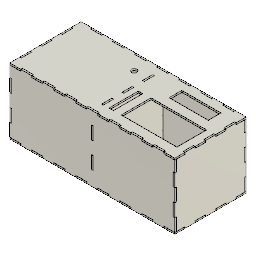
Final Enclosure (Autodesk Fusion 360 design; units mm, degrees)
Autodesk Fusion 360 part; units mm, degrees
note: some values were not read from the file. Chosen so that the rebuilt part matches the saved one: which bodies a step acts on.
(part 1 of 2)
sketch "Bottom Panel Profile Sketch" plane through (0, 0, 0) normal (0, 0, 1) x (1, 0, 0) in component "Main Box"
  line L0 (0, 0) -> (300, 0)
  line L1 (300, 0) -> (300, 130)
  line L2 (300, 130) -> (0, 130)
  line L3 (0, 130) -> (0, 0)
  dimension "d21" = 300
  dimension "d22" = 130
  constraint horizontal L0
  constraint vertical L1
  constraint horizontal L2
  constraint vertical L3
  constraint coincident L0.start L3.end
  measures "d21" distance of L0.start L0.end
  measures "d22" distance of L0.start L2.end
extrude "Bottom Panel Extrude" add sketch "Bottom Panel Profile Sketch" along normal blind 3 makes body 1 in component "Main Box"
sketch "Bottom Panel Front Fingers Sketch" plane through (0, 0, 0) normal (0, -1, 0) x (1, 0, 0) in component "Main Box"
  line L0 (0, 0) -> (300, 0)
  line L1 (300, 0) -> (300, 3)
  line L2 (300, 3) -> (0, 3)
  line L3 (0, 3) -> (0, 0)
  line L4 (150, 3) -> (150, 0) construction
  line L5 (20, 1.5) -> (280, 1.5) construction
  line L6 (20, 0) -> (40, 0)
  line L7 (40, 0) -> (40, 3)
  line L8 (40, 3) -> (20, 3)
  line L9 (20, 3) -> (20, 0)
  dimension "d25" = 20
  dimension "d26" = 260
  constraint midpoint L2 L4.start
  constraint midpoint L0 L4.end
  constraint perpendicular L4 L5
  constraint midpoint L4 L5
  constraint horizontal L6
  constraint vertical L7
  constraint horizontal L8
  constraint vertical L9
  constraint coincident L2 L7.end
  constraint coincident L0 L6.start
  constraint coincident L5.start L9
  measures "d25" horizontal distance of L7.end L8.end
  measures "d26" horizontal distance of L5.start L5.end
extrude "Bottom Panel Front Finger Extrude" cut sketch "Bottom Panel Front Fingers Sketch" against normal blind 3 contours L0 L2 L6 L7 L8 L9 bodies 1 in component "Main Box"
pattern_linear "Bottom Panel Length Fingers Pattern" count 7 spacing 40 along (1, 0, 0) count 2 spacing 127 along (0, 1, 0) of "Bottom Panel Front Finger Extrude" in component "Main Box"
sketch "Bottom Panel Left Fingers Sketch" plane through (0, 0, 0) normal (-1, 0, 0) x (0, -1, 0) in component "Main Box"
  line L0 (-130, 0) -> (0, 0)
  line L1 (0, 0) -> (0, 3)
  line L2 (0, 3) -> (-130, 3)
  line L3 (-130, 3) -> (-130, 0)
  line L4 (-65, 3) -> (-65, 0) construction
  line L5 (-111.4286, 1.5) -> (-18.5714, 1.5) construction
  line L6 (-18.5714, 0) -> (-37.1429, 0)
  line L7 (-37.1429, 0) -> (-37.1429, 3)
  line L8 (-37.1429, 3) -> (-18.5714, 3)
  line L9 (-18.5714, 3) -> (-18.5714, 0)
  dimension "d33" = 18.5714
  dimension "d34" = 92.8571
  constraint midpoint L2 L4.start
  constraint midpoint L0 L4.end
  constraint perpendicular L4 L5
  constraint midpoint L4 L5
  constraint horizontal L6
  constraint vertical L7
  constraint horizontal L8
  constraint vertical L9
  constraint coincident L2 L7.end
  constraint coincident L0 L6.start
  constraint coincident L5.end L9
  measures "d33" horizontal distance of L6.start L6.end
  measures "d34" horizontal distance of L5.start L5.end
extrude "Bottom Panel Left Finger Extrude" cut sketch "Bottom Panel Left Fingers Sketch" against normal blind 3 contours L0 L2 L6 L7 L8 L9 bodies 1 in component "Main Box"
pattern_linear "Bottom Panel Width Fingers Pattern" count 3 spacing 37.1429 along (0, 1, 0) count 3 spacing 148.5 along (1, 0, 0) of "Bottom Panel Left Finger Extrude" in component "Main Box"
sketch "Front Panel Profile Sketch" plane through (0, 0, 0) normal (0, 1, 0) x (1, 0, 0) in component "Main Box"
  line L0 (0, 0) -> (300, 0)
  line L1 (300, 0) -> (300, -120)
  line L2 (300, -120) -> (0, -120)
  line L3 (0, -120) -> (0, 0)
  dimension "d41" = 300
  dimension "d42" = 120
  constraint horizontal L0
  constraint vertical L1
  constraint horizontal L2
  constraint vertical L3
  constraint coincident L0.start L3.end
  measures "d41" distance of L0.start L0.end
  measures "d42" distance of L0.start L2.end
extrude "Front Panel Extrude" add sketch "Front Panel Profile Sketch" along normal blind 3 separate body makes body 2 in component "Main Box"
combine "Front Panel Combine" operation cut target body 2 tool bodies 1 keep tools in component "Main Box"
sketch "Front Panel Left Fingers Sketch" plane through (0, 0, 0) normal (0, -1, 0) x (1, 0, 0) in component "Main Box"
  line L0 (300, 3) -> (300, 120)
  line L1 (300, 120) -> (0, 120)
  line L2 (0, 120) -> (0, 3)
  line L3 (280, 3) -> (300, 3)
  line L4 (20, 3) -> (20, 0)
  line L5 (20, 0) -> (40, 0)
  line L6 (40, 0) -> (40, 3)
  line L7 (40, 3) -> (60, 3)
  line L8 (0, 61.5) -> (3, 61.5) construction
  line L9 (1.5, 96.6) -> (1.5, 26.4) construction
  line L10 (0, 26.4) -> (3, 26.4)
  line L11 (3, 26.4) -> (3, 49.8)
  line L12 (3, 49.8) -> (0, 49.8)
  line L13 (0, 49.8) -> (0, 26.4)
  line L14 (60, 3) -> (60, 0)
  line L15 (60, 0) -> (80, 0)
  line L16 (80, 0) -> (80, 3)
  line L17 (80, 3) -> (100, 3)
  line L18 (100, 3) -> (100, 0)
  line L19 (100, 0) -> (120, 0)
  line L20 (120, 0) -> (120, 3)
  line L21 (120, 3) -> (140, 3)
  line L22 (140, 3) -> (140, 0)
  line L23 (140, 0) -> (160, 0)
  line L24 (160, 0) -> (160, 3)
  line L25 (160, 3) -> (180, 3)
  line L26 (180, 3) -> (180, 0)
  line L27 (180, 0) -> (200, 0)
  line L28 (200, 0) -> (200, 3)
  line L29 (200, 3) -> (220, 3)
  line L30 (220, 3) -> (220, 0)
  line L31 (220, 0) -> (240, 0)
  line L32 (240, 0) -> (240, 3)
  line L33 (240, 3) -> (260, 3)
  line L34 (260, 3) -> (260, 0)
  line L35 (260, 0) -> (280, 0)
  line L36 (280, 0) -> (280, 3)
  line L37 (0, 3) -> (20, 3)
  dimension "d45" = 3
  dimension "d46" = 23.4
  dimension "d47" = 70.2
  constraint midpoint L2 L8.start
  constraint perpendicular L2 L8
  constraint perpendicular L8 L9
  constraint midpoint L8 L9
  constraint horizontal L10
  constraint vertical L11
  constraint horizontal L12
  constraint vertical L13
  constraint coincident L2 L10.start
  constraint coincident L9.end L10
  constraint coincident L8.end L11
  measures "d45" distance of L8.start L8.end
  measures "d46" vertical distance of L10.start L12.end
  measures "d47" vertical distance of L9.start L9.end
extrude "Front Panel Left Fingers Extrude" cut sketch "Front Panel Left Fingers Sketch" against normal blind 3 contours L2 L10 L11 L12 L13 bodies 2 in component "Main Box"
pattern_linear "Front Panel Height Fingers Pattern" count 2 spacing 46.8 along (0, 0, 1) count 3 spacing 148.5 along (1, 0, 0) of "Front Panel Left Fingers Extrude" in component "Main Box"
pattern_linear "Front Panel Pattern" count 2 spacing 127 along (0, 1, 0) of bodies 2 makes body 3 in component "Main Box"
sketch "Left Panel Profile Sketch" plane through (0, 0, 0) normal (1, 0, 0) x (0, 1, 0) in component "Main Box"
  line L0 (0, 0) -> (130, 0)
  line L1 (130, 0) -> (130, 120)
  line L2 (130, 120) -> (0, 120)
  line L3 (0, 120) -> (0, 0)
  dimension "d58" = 130
  dimension "d59" = 120
  constraint horizontal L0
  constraint vertical L1
  constraint horizontal L2
  constraint vertical L3
  constraint coincident L0.start L3.end
  measures "d58" distance of L0.start L0.end
  measures "d59" distance of L0.start L2.end
extrude "Left Panel Extrude" add sketch "Left Panel Profile Sketch" along normal blind 3 separate body makes body 4 in component "Main Box"
sketch "Left Panel Front Fingers Sketch" plane through (0, 0, 0) normal (0, -1, 0) x (1, 0, 0) in component "Main Box"
  line L0 (0, 120) -> (0, 0)
  line L1 (0, 0) -> (3, 0)
  line L2 (3, 0) -> (3, 120)
  line L3 (3, 120) -> (0, 120)
  line L4 (0, 120) -> (3, 120)
  line L5 (3, 120) -> (3, 96.6)
  line L6 (3, 96.6) -> (0, 96.6)
  line L7 (0, 96.6) -> (0, 120)
  dimension "d72" = 23.4
  constraint horizontal L4
  constraint vertical L5
  constraint horizontal L6
  constraint vertical L7
  constraint coincident L2 L5.end
  constraint coincident L0.start L3.end
  measures "d72" vertical distance of L0.start L6.end
extrude "Left Panel Front Fingers Extrude" cut sketch "Left Panel Front Fingers Sketch" against normal blind 3 contours L0 L2 L3 L4 L5 L6 L7 bodies 4 in component "Main Box"
pattern_linear "Left Panel Slots Pattern" count 2 spacing 127 along (0, 1, 0) of "Left Panel Front Fingers Extrude" in component "Main Box"
combine "Left Panel Combine" operation cut target body 4 tool bodies 3 1 2 keep tools in component "Main Box"
pattern_linear "Left Panel Pattern" count 3 spacing 148.5 along (1, 0, 0) of bodies 4 makes body 5 at (300, 61.9048, 49.8) makes body 6 at (151.5, 61.9048, 49.8) in component "Main Box"
sketch "Sketch1" plane through (0, 0, 0) normal (0, -1, 0) x (1, 0, 0)
  line L0 (297, 49.8) -> (300, 49.8)
  line L1 (300, 96.6) -> (300, 120)
  line L2 (300, 120) -> (0, 120)
  line L3 (0, 120) -> (0, 96.6)
  line L4 (0, 49.8) -> (3, 49.8)
  line L5 (3, 49.8) -> (3, 26.4)
  line L6 (3, 26.4) -> (0, 26.4)
  line L7 (0, 26.4) -> (0, 3)
  line L8 (0, 3) -> (20, 3)
  line L9 (20, 3) -> (20, 0)
  line L10 (20, 0) -> (40, 0)
  line L11 (40, 0) -> (40, 3)
  line L12 (40, 3) -> (60, 3)
  line L13 (60, 3) -> (60, 0)
  line L14 (60, 0) -> (80, 0)
  line L15 (80, 0) -> (80, 3)
  line L16 (80, 3) -> (100, 3)
  line L17 (100, 3) -> (100, 0)
  line L18 (100, 0) -> (120, 0)
  line L19 (120, 0) -> (120, 3)
  line L20 (120, 3) -> (140, 3)
  line L21 (140, 3) -> (140, 0)
  line L22 (140, 0) -> (160, 0)
  line L23 (160, 0) -> (160, 3)
  line L24 (160, 3) -> (180, 3)
  line L25 (180, 3) -> (180, 0)
  line L26 (180, 0) -> (200, 0)
  line L27 (200, 0) -> (200, 3)
  line L28 (200, 3) -> (220, 3)
  line L29 (220, 3) -> (220, 0)
  line L30 (220, 0) -> (240, 0)
  line L31 (240, 0) -> (240, 3)
  line L32 (240, 3) -> (260, 3)
  line L33 (260, 3) -> (260, 0)
  line L34 (260, 0) -> (280, 0)
  line L35 (280, 0) -> (280, 3)
  line L36 (280, 3) -> (300, 3)
  line L37 (300, 3) -> (300, 26.4)
  line L38 (300, 26.4) -> (297, 26.4)
  line L39 (297, 26.4) -> (297, 49.8)
  line L40 (151.5, 26.4) -> (148.5, 26.4)
  line L41 (148.5, 26.4) -> (148.5, 49.8)
  line L42 (148.5, 49.8) -> (151.5, 49.8)
  line L43 (151.5, 49.8) -> (151.5, 26.4)
  line L44 (297, 96.6) -> (300, 96.6)
  line L45 (0, 96.6) -> (3, 96.6)
  line L46 (3, 96.6) -> (3, 73.2)
  line L47 (3, 73.2) -> (0, 73.2)
  line L48 (0, 73.2) -> (0, 49.8)
  line L49 (300, 49.8) -> (300, 73.2)
  line L50 (300, 73.2) -> (297, 73.2)
  line L51 (297, 73.2) -> (297, 96.6)
  line L52 (151.5, 73.2) -> (148.5, 73.2)
  line L53 (148.5, 96.6) -> (151.5, 96.6)
extrude "Extrude1" add 1 faces at (102.8333, 68.0952, 3) along direction (0, 0, 1) blind 117 separate body on bodies 1 makes body 7
extrude "Extrude2" add 1 faces at (102.8333, 68.0952, 3) along direction (0, 0, 1) blind 3 from surface at 114 separate body on bodies 1 makes body 8
combine "Combine3" operation cut target body 4 tool bodies 8 keep tools in component "Main Box"
combine "Combine4" operation cut target body 2 tool bodies 8 keep tools in component "Main Box"
combine "Combine5" operation cut target body 5 tool bodies 8 keep tools in component "Main Box"
combine "Combine6" operation cut target body 3 tool bodies 8 keep tools in component "Main Box"
combine "Combine7" operation cut target body 6 tool bodies 8 keep tools in component "Main Box"
sketch "Sketch12" plane through (0, 0, 120) normal (0, 0, 1) x (-1, 0, 0)
  line L0 (-151.5, -18.5714) -> (-148.5, -18.5714)
  line L1 (-148.5, -18.5714) -> (-148.5, -37.1429)
  line L2 (-148.5, -37.1429) -> (-151.5, -37.1429)
  line L3 (-151.5, -37.1429) -> (-151.5, -18.5714)
  line L4 (-151.5, -55.7143) -> (-148.5, -55.7143)
  line L5 (-148.5, -55.7143) -> (-148.5, -74.2857)
  line L6 (-148.5, -74.2857) -> (-151.5, -74.2857)
  line L7 (-151.5, -74.2857) -> (-151.5, -55.7143)
  line L8 (-151.5, -92.8571) -> (-148.5, -92.8571)
  line L9 (-148.5, -92.8571) -> (-148.5, -111.4286)
  line L10 (-148.5, -111.4286) -> (-151.5, -111.4286)
  line L11 (-151.5, -111.4286) -> (-151.5, -92.8571)
  line L12 (-300, -92.8571) -> (-297, -92.8571)
  line L13 (-297, -92.8571) -> (-297, -111.4286)
  line L14 (-297, -111.4286) -> (-300, -111.4286)
  line L15 (-300, -111.4286) -> (-300, -130)
  line L16 (-300, -130) -> (-280, -130)
  line L17 (-280, -130) -> (-280, -127)
  line L18 (-280, -127) -> (-260, -127)
  line L19 (-260, -127) -> (-260, -130)
  line L20 (-260, -130) -> (-240, -130)
  line L21 (-240, -130) -> (-240, -127)
  line L22 (-240, -127) -> (-220, -127)
  line L23 (-220, -127) -> (-220, -130)
  line L24 (-220, -130) -> (-200, -130)
  line L25 (-200, -130) -> (-200, -127)
  line L26 (-200, -127) -> (-180, -127)
  line L27 (-180, -127) -> (-180, -130)
  line L28 (-180, -130) -> (-160, -130)
  line L29 (-160, -130) -> (-160, -127)
  line L30 (-160, -127) -> (-140, -127)
  line L31 (-140, -127) -> (-140, -130)
  line L32 (-140, -130) -> (-120, -130)
  line L33 (-120, -130) -> (-120, -127)
  line L34 (-120, -127) -> (-100, -127)
  line L35 (-100, -127) -> (-100, -130)
  line L36 (-100, -130) -> (-80, -130)
  line L37 (-80, -130) -> (-80, -127)
  line L38 (-80, -127) -> (-60, -127)
  line L39 (-60, -127) -> (-60, -130)
  line L40 (-60, -130) -> (-40, -130)
  line L41 (-40, -130) -> (-40, -127)
  line L42 (-40, -127) -> (-20, -127)
  line L43 (-20, -127) -> (-20, -130)
  line L44 (-20, -130) -> (0, -130)
  line L45 (0, -130) -> (0, -111.4286)
  line L46 (0, -111.4286) -> (-3, -111.4286)
  line L47 (-3, -111.4286) -> (-3, -92.8571)
  line L48 (-3, -92.8571) -> (0, -92.8571)
  line L49 (0, -92.8571) -> (0, -74.2857)
  line L50 (0, -74.2857) -> (-3, -74.2857)
  line L51 (-3, -74.2857) -> (-3, -55.7143)
  line L52 (-3, -55.7143) -> (0, -55.7143)
  line L53 (0, -55.7143) -> (0, -37.1429)
  line L54 (0, -37.1429) -> (-3, -37.1429)
  line L55 (-3, -37.1429) -> (-3, -18.5714)
  line L56 (-3, -18.5714) -> (0, -18.5714)
  line L57 (0, -18.5714) -> (0, 0)
  line L58 (0, 0) -> (-20, 0)
  line L59 (-20, 0) -> (-20, -3)
  line L60 (-20, -3) -> (-40, -3)
  line L61 (-40, -3) -> (-40, 0)
  line L62 (-40, 0) -> (-60, 0)
  line L63 (-60, 0) -> (-60, -3)
  line L64 (-60, -3) -> (-80, -3)
  line L65 (-80, -3) -> (-80, 0)
  line L66 (-80, 0) -> (-100, 0)
  line L67 (-100, 0) -> (-100, -3)
  line L68 (-100, -3) -> (-120, -3)
  line L69 (-120, -3) -> (-120, 0)
  line L70 (-120, 0) -> (-140, 0)
  line L71 (-140, 0) -> (-140, -3)
  line L72 (-140, -3) -> (-160, -3)
  line L73 (-160, -3) -> (-160, 0)
  line L74 (-160, 0) -> (-180, 0)
  line L75 (-180, 0) -> (-180, -3)
  line L76 (-180, -3) -> (-200, -3)
  line L77 (-200, -3) -> (-200, 0)
  line L78 (-200, 0) -> (-220, 0)
  line L79 (-220, 0) -> (-220, -3)
  line L80 (-220, -3) -> (-240, -3)
  line L81 (-240, -3) -> (-240, 0)
  line L82 (-240, 0) -> (-260, 0)
  line L83 (-260, 0) -> (-260, -3)
  line L84 (-260, -3) -> (-280, -3)
  line L85 (-280, -3) -> (-280, 0)
  line L86 (-280, 0) -> (-300, 0)
  line L87 (-300, 0) -> (-300, -18.5714)
  line L88 (-300, -18.5714) -> (-297, -18.5714)
  line L89 (-297, -18.5714) -> (-297, -37.1429)
  line L90 (-297, -37.1429) -> (-300, -37.1429)
  line L91 (-300, -37.1429) -> (-300, -55.7143)
  line L92 (-300, -55.7143) -> (-297, -55.7143)
  line L93 (-297, -55.7143) -> (-297, -74.2857)
  line L94 (-297, -74.2857) -> (-300, -74.2857)
  line L95 (-300, -74.2857) -> (-300, -92.8571)
  circle A0 centre (-125.8569, -100.5311) radius 5
  line L96 (-199.7569, -113.0322) -> (-270.7569, -113.0322)
  line L97 (-270.7569, -113.0322) -> (-270.7569, -90.0322)
  line L98 (-270.7569, -90.0322) -> (-199.7569, -90.0322)
  line L99 (-199.7569, -90.0322) -> (-199.7569, -113.0322)
  line L100 (-183.4296, -73.3855) -> (-284.4296, -73.3855)
  line L101 (-284.4296, -73.3855) -> (-284.4296, -19.3855)
  line L102 (-284.4296, -19.3855) -> (-183.4296, -19.3855)
  line L103 (-183.4296, -19.3855) -> (-183.4296, -73.3855)
  line L104 (-161.4021, -72.4445) -> (-169.4021, -72.4445)
  line L105 (-169.4021, -72.4445) -> (-169.4021, -19.1021)
  line L106 (-169.4021, -19.1021) -> (-161.4021, -19.1021)
  line L107 (-161.4021, -19.1021) -> (-161.4021, -72.4445)
  dimension "d109" = 10
  dimension "d110" = 71
  dimension "d111" = 23
  dimension "d112" = 101
  dimension "d113" = 54
  dimension "d114" = 8
  constraint horizontal L96
  constraint vertical L97
  constraint horizontal L98
  constraint vertical L99
  constraint horizontal L100
  constraint vertical L101
  constraint horizontal L102
  constraint vertical L103
  constraint horizontal L104
  constraint vertical L105
  constraint horizontal L106
  constraint vertical L107
  measures "d109" diameter of A0
  measures "d110" distance of L96.start L96.end
  measures "d111" distance of L96.start L98.end
  measures "d112" distance of L100.start L100.end
  measures "d113" distance of L100.start L102.end
  measures "d114" distance of L104.start L104.end
extrude "Extrude4" cut sketch "Sketch12" against normal blind 3 contours A0 | L96 L97 L98 L99 | L100 L101 L102 L103 | L104 L105 L106 L107 bodies 8
sketch "Sketch14" plane through (151.5, 0, 0) normal (1, 0, 0) x (0, 1, 0)
  line L0 (18.5714, 117) -> (3, 117)
  line L1 (3, 117) -> (3, 96.6)
  line L2 (3, 96.6) -> (0, 96.6)
  line L3 (0, 96.6) -> (0, 73.2)
  line L4 (0, 73.2) -> (3, 73.2)
  line L5 (3, 73.2) -> (3, 49.8)
  line L6 (3, 49.8) -> (0, 49.8)
  line L7 (0, 49.8) -> (0, 26.4)
  line L8 (0, 26.4) -> (3, 26.4)
  line L9 (3, 26.4) -> (3, 3)
  line L10 (3, 3) -> (18.5714, 3)
  line L11 (18.5714, 3) -> (18.5714, 0)
  line L12 (18.5714, 0) -> (37.1429, 0)
  line L13 (37.1429, 0) -> (37.1429, 3)
  line L14 (37.1429, 3) -> (55.7143, 3)
  line L15 (55.7143, 3) -> (55.7143, 0)
  line L16 (55.7143, 0) -> (74.2857, 0)
  line L17 (74.2857, 0) -> (74.2857, 3)
  line L18 (74.2857, 3) -> (92.8571, 3)
  line L19 (92.8571, 3) -> (92.8571, 0)
  line L20 (92.8571, 0) -> (111.4286, 0)
  line L21 (111.4286, 0) -> (111.4286, 3)
  line L22 (111.4286, 3) -> (127, 3)
  line L23 (127, 3) -> (127, 26.4)
  line L24 (127, 26.4) -> (130, 26.4)
  line L25 (130, 26.4) -> (130, 49.8)
  line L26 (130, 49.8) -> (127, 49.8)
  line L27 (127, 49.8) -> (127, 73.2)
  line L28 (127, 73.2) -> (130, 73.2)
  line L29 (130, 73.2) -> (130, 96.6)
  line L30 (130, 96.6) -> (127, 96.6)
  line L31 (127, 96.6) -> (127, 117)
  line L32 (127, 117) -> (111.4286, 117)
  line L33 (111.4286, 117) -> (111.4286, 120)
  line L34 (111.4286, 120) -> (92.8571, 120)
  line L35 (92.8571, 120) -> (92.8571, 117)
  line L36 (92.8571, 117) -> (74.2857, 117)
  line L37 (74.2857, 117) -> (74.2857, 120)
  line L38 (74.2857, 120) -> (55.7143, 120)
  line L39 (55.7143, 120) -> (55.7143, 117)
  line L40 (55.7143, 117) -> (37.1429, 117)
  line L41 (37.1429, 117) -> (37.1429, 120)
  line L42 (37.1429, 120) -> (18.5714, 120)
  line L43 (18.5714, 120) -> (18.5714, 117)
  circle A0 centre (63.791, 90.8075) radius 9.4231
extrude "Extrude10" [rolled back] taper angle 0 in component "Main Box"
sketch "FRONTBACK" plane through (0, 130, 0) normal (0, 1, 0) x (-1, 0, 0)
  line L0 (0, 117) -> (-20, 117)
  line L1 (-20, 117) -> (-20, 120)
  line L2 (-20, 120) -> (-40, 120)
  line L3 (-40, 120) -> (-40, 117)
  line L4 (-40, 117) -> (-60, 117)
  line L5 (-60, 117) -> (-60, 120)
  line L6 (-60, 120) -> (-80, 120)
  line L7 (-80, 120) -> (-80, 117)
  line L8 (-80, 117) -> (-100, 117)
  line L9 (-100, 117) -> (-100, 120)
  line L10 (-100, 120) -> (-120, 120)
  line L11 (-120, 120) -> (-120, 117)
  line L12 (-120, 117) -> (-140, 117)
  line L13 (-140, 117) -> (-140, 120)
  line L14 (-140, 120) -> (-160, 120)
  line L15 (-160, 120) -> (-160, 117)
  line L16 (-160, 117) -> (-180, 117)
  line L17 (-180, 117) -> (-180, 120)
  line L18 (-180, 120) -> (-200, 120)
  line L19 (-200, 120) -> (-200, 117)
  line L20 (-200, 117) -> (-220, 117)
  line L21 (-220, 117) -> (-220, 120)
  line L22 (-220, 120) -> (-240, 120)
  line L23 (-240, 120) -> (-240, 117)
  line L24 (-240, 117) -> (-260, 117)
  line L25 (-260, 117) -> (-260, 120)
  line L26 (-260, 120) -> (-280, 120)
  line L27 (-280, 120) -> (-280, 117)
  line L28 (-280, 117) -> (-300, 117)
  line L29 (-300, 117) -> (-300, 96.6)
  line L30 (-300, 96.6) -> (-297, 96.6)
  line L31 (-297, 96.6) -> (-297, 73.2)
  line L32 (-297, 73.2) -> (-300, 73.2)
  line L33 (-300, 73.2) -> (-300, 49.8)
  line L34 (-300, 49.8) -> (-297, 49.8)
  line L35 (-297, 49.8) -> (-297, 26.4)
  line L36 (-297, 26.4) -> (-300, 26.4)
  line L37 (-300, 26.4) -> (-300, 3)
  line L38 (-300, 3) -> (-280, 3)
  line L39 (-280, 3) -> (-280, 0)
  line L40 (-280, 0) -> (-260, 0)
  line L41 (-260, 0) -> (-260, 3)
  line L42 (-260, 3) -> (-240, 3)
  line L43 (-240, 3) -> (-240, 0)
  line L44 (-240, 0) -> (-220, 0)
  line L45 (-220, 0) -> (-220, 3)
  line L46 (-220, 3) -> (-200, 3)
  line L47 (-200, 3) -> (-200, 0)
  line L48 (-200, 0) -> (-180, 0)
  line L49 (-180, 0) -> (-180, 3)
  line L50 (-180, 3) -> (-160, 3)
  line L51 (-160, 3) -> (-160, 0)
  line L52 (-160, 0) -> (-140, 0)
  line L53 (-140, 0) -> (-140, 3)
  line L54 (-140, 3) -> (-120, 3)
  line L55 (-120, 3) -> (-120, 0)
  line L56 (-120, 0) -> (-100, 0)
  line L57 (-100, 0) -> (-100, 3)
  line L58 (-100, 3) -> (-80, 3)
  line L59 (-80, 3) -> (-80, 0)
  line L60 (-80, 0) -> (-60, 0)
  line L61 (-60, 0) -> (-60, 3)
  line L62 (-60, 3) -> (-40, 3)
  line L63 (-40, 3) -> (-40, 0)
  line L64 (-40, 0) -> (-20, 0)
  line L65 (-20, 0) -> (-20, 3)
  line L66 (-20, 3) -> (0, 3)
  line L67 (0, 3) -> (0, 26.4)
  line L68 (0, 26.4) -> (-3, 26.4)
  line L69 (-3, 26.4) -> (-3, 49.8)
  line L70 (-3, 49.8) -> (0, 49.8)
  line L71 (0, 49.8) -> (0, 73.2)
  line L72 (0, 73.2) -> (-3, 73.2)
  line L73 (-3, 73.2) -> (-3, 96.6)
  line L74 (-3, 96.6) -> (0, 96.6)
  line L75 (0, 96.6) -> (0, 117)
  line L76 (-148.5, 73.2) -> (-151.5, 73.2)
  line L77 (-151.5, 73.2) -> (-151.5, 96.6)
  line L78 (-151.5, 96.6) -> (-148.5, 96.6)
  line L79 (-148.5, 96.6) -> (-148.5, 73.2)
  line L80 (-148.5, 26.4) -> (-151.5, 26.4)
  line L81 (-151.5, 26.4) -> (-151.5, 49.8)
  line L82 (-151.5, 49.8) -> (-148.5, 49.8)
  line L83 (-148.5, 49.8) -> (-148.5, 26.4)
sketch "LEFT RIGHT" plane through (300, 0, 0) normal (1, 0, 0) x (0, 1, 0)
  line L0 (18.5714, 117) -> (3, 117)
  line L1 (3, 117) -> (3, 96.6)
  line L2 (3, 96.6) -> (0, 96.6)
  line L3 (0, 96.6) -> (0, 73.2)
  line L4 (0, 73.2) -> (3, 73.2)
  line L5 (3, 73.2) -> (3, 49.8)
  line L6 (3, 49.8) -> (0, 49.8)
  line L7 (0, 49.8) -> (0, 26.4)
  line L8 (0, 26.4) -> (3, 26.4)
  line L9 (3, 26.4) -> (3, 3)
  line L10 (3, 3) -> (18.5714, 3)
  line L11 (18.5714, 3) -> (18.5714, 0)
  line L12 (18.5714, 0) -> (37.1429, 0)
  line L13 (37.1429, 0) -> (37.1429, 3)
  line L14 (37.1429, 3) -> (55.7143, 3)
  line L15 (55.7143, 3) -> (55.7143, 0)
  line L16 (55.7143, 0) -> (74.2857, 0)
  line L17 (74.2857, 0) -> (74.2857, 3)
  line L18 (74.2857, 3) -> (92.8571, 3)
  line L19 (92.8571, 3) -> (92.8571, 0)
  line L20 (92.8571, 0) -> (111.4286, 0)
  line L21 (111.4286, 0) -> (111.4286, 3)
  line L22 (111.4286, 3) -> (127, 3)
  line L23 (127, 3) -> (127, 26.4)
  line L24 (127, 26.4) -> (130, 26.4)
  line L25 (130, 26.4) -> (130, 49.8)
  line L26 (130, 49.8) -> (127, 49.8)
  line L27 (127, 49.8) -> (127, 73.2)
  line L28 (127, 73.2) -> (130, 73.2)
  line L29 (130, 73.2) -> (130, 96.6)
  line L30 (130, 96.6) -> (127, 96.6)
  line L31 (127, 96.6) -> (127, 117)
  line L32 (127, 117) -> (111.4286, 117)
  line L33 (111.4286, 117) -> (111.4286, 120)
  line L34 (111.4286, 120) -> (92.8571, 120)
  line L35 (92.8571, 120) -> (92.8571, 117)
  line L36 (92.8571, 117) -> (74.2857, 117)
  line L37 (74.2857, 117) -> (74.2857, 120)
  line L38 (74.2857, 120) -> (55.7143, 120)
  line L39 (55.7143, 120) -> (55.7143, 117)
  line L40 (55.7143, 117) -> (37.1429, 117)
  line L41 (37.1429, 117) -> (37.1429, 120)
  line L42 (37.1429, 120) -> (18.5714, 120)
  line L43 (18.5714, 120) -> (18.5714, 117)
sketch "MIDDLE PIECE" plane through (151.5, 0, 0) normal (1, 0, 0) x (0, 1, 0)
  circle A0 centre (63.791, 90.8075) radius 9.4231
  line L0 (18.5714, 117) -> (3, 117)
  line L1 (3, 117) -> (3, 96.6)
  line L2 (3, 96.6) -> (0, 96.6)
  line L3 (0, 96.6) -> (0, 73.2)
  line L4 (0, 73.2) -> (3, 73.2)
  line L5 (3, 73.2) -> (3, 49.8)
  line L6 (3, 49.8) -> (0, 49.8)
  line L7 (0, 49.8) -> (0, 26.4)
  line L8 (0, 26.4) -> (3, 26.4)
  line L9 (3, 26.4) -> (3, 3)
  line L10 (3, 3) -> (18.5714, 3)
  line L11 (18.5714, 3) -> (18.5714, 0)
  line L12 (18.5714, 0) -> (37.1429, 0)
  line L13 (37.1429, 0) -> (37.1429, 3)
  line L14 (37.1429, 3) -> (55.7143, 3)
  line L15 (55.7143, 3) -> (55.7143, 0)
  line L16 (55.7143, 0) -> (74.2857, 0)
  line L17 (74.2857, 0) -> (74.2857, 3)
  line L18 (74.2857, 3) -> (92.8571, 3)
  line L19 (92.8571, 3) -> (92.8571, 0)
  line L20 (92.8571, 0) -> (111.4286, 0)
  line L21 (111.4286, 0) -> (111.4286, 3)
  line L22 (111.4286, 3) -> (127, 3)
  line L23 (127, 3) -> (127, 26.4)
  line L24 (127, 26.4) -> (130, 26.4)
  line L25 (130, 26.4) -> (130, 49.8)
  line L26 (130, 49.8) -> (127, 49.8)
  line L27 (127, 49.8) -> (127, 73.2)
  line L28 (127, 73.2) -> (130, 73.2)
  line L29 (130, 73.2) -> (130, 96.6)
  line L30 (130, 96.6) -> (127, 96.6)
  line L31 (127, 96.6) -> (127, 117)
  line L32 (127, 117) -> (111.4286, 117)
  line L33 (111.4286, 117) -> (111.4286, 120)
  line L34 (111.4286, 120) -> (92.8571, 120)
  line L35 (92.8571, 120) -> (92.8571, 117)
  line L36 (92.8571, 117) -> (74.2857, 117)
  line L37 (74.2857, 117) -> (74.2857, 120)
  line L38 (74.2857, 120) -> (55.7143, 120)
  line L39 (55.7143, 120) -> (55.7143, 117)
  line L40 (55.7143, 117) -> (37.1429, 117)
  line L41 (37.1429, 117) -> (37.1429, 120)
  line L42 (37.1429, 120) -> (18.5714, 120)
  line L43 (18.5714, 120) -> (18.5714, 117)
sketch "BOTTOM" plane through (0, 0, 3) normal (0, 0, 1) x (-1, 0, 0)
  line L0 (-151.5, -18.5714) -> (-148.5, -18.5714)
  line L1 (-148.5, -18.5714) -> (-148.5, -37.1429)
  line L2 (-148.5, -37.1429) -> (-151.5, -37.1429)
  line L3 (-151.5, -37.1429) -> (-151.5, -18.5714)
  line L4 (-151.5, -55.7143) -> (-148.5, -55.7143)
  line L5 (-148.5, -55.7143) -> (-148.5, -74.2857)
  line L6 (-148.5, -74.2857) -> (-151.5, -74.2857)
  line L7 (-151.5, -74.2857) -> (-151.5, -55.7143)
  line L8 (-151.5, -92.8571) -> (-148.5, -92.8571)
  line L9 (-148.5, -92.8571) -> (-148.5, -111.4286)
  line L10 (-148.5, -111.4286) -> (-151.5, -111.4286)
  line L11 (-151.5, -111.4286) -> (-151.5, -92.8571)
  line L12 (-300, -92.8571) -> (-297, -92.8571)
  line L13 (-297, -92.8571) -> (-297, -111.4286)
  line L14 (-297, -111.4286) -> (-300, -111.4286)
  line L15 (-300, -111.4286) -> (-300, -130)
  line L16 (-300, -130) -> (-280, -130)
  line L17 (-280, -130) -> (-280, -127)
  line L18 (-280, -127) -> (-260, -127)
  line L19 (-260, -127) -> (-260, -130)
  line L20 (-260, -130) -> (-240, -130)
  line L21 (-240, -130) -> (-240, -127)
  line L22 (-240, -127) -> (-220, -127)
  line L23 (-220, -127) -> (-220, -130)
  line L24 (-220, -130) -> (-200, -130)
  line L25 (-200, -130) -> (-200, -127)
  line L26 (-200, -127) -> (-180, -127)
  line L27 (-180, -127) -> (-180, -130)
  line L28 (-180, -130) -> (-160, -130)
  line L29 (-160, -130) -> (-160, -127)
  line L30 (-160, -127) -> (-140, -127)
  line L31 (-140, -127) -> (-140, -130)
  line L32 (-140, -130) -> (-120, -130)
  line L33 (-120, -130) -> (-120, -127)
  line L34 (-120, -127) -> (-100, -127)
  line L35 (-100, -127) -> (-100, -130)
  line L36 (-100, -130) -> (-80, -130)
  line L37 (-80, -130) -> (-80, -127)
  line L38 (-80, -127) -> (-60, -127)
  line L39 (-60, -127) -> (-60, -130)
  line L40 (-60, -130) -> (-40, -130)
  line L41 (-40, -130) -> (-40, -127)
  line L42 (-40, -127) -> (-20, -127)
  line L43 (-20, -127) -> (-20, -130)
  line L44 (-20, -130) -> (0, -130)
  line L45 (0, -130) -> (0, -111.4286)
  line L46 (0, -111.4286) -> (-3, -111.4286)
  line L47 (-3, -111.4286) -> (-3, -92.8571)
  line L48 (-3, -92.8571) -> (0, -92.8571)
  line L49 (0, -92.8571) -> (0, -74.2857)
  line L50 (0, -74.2857) -> (-3, -74.2857)
  line L51 (-3, -74.2857) -> (-3, -55.7143)
  line L52 (-3, -55.7143) -> (0, -55.7143)
  line L53 (0, -55.7143) -> (0, -37.1429)
  line L54 (0, -37.1429) -> (-3, -37.1429)
  line L55 (-3, -37.1429) -> (-3, -18.5714)
  line L56 (-3, -18.5714) -> (0, -18.5714)
  line L57 (0, -18.5714) -> (0, 0)
  line L58 (0, 0) -> (-20, 0)
  line L59 (-20, 0) -> (-20, -3)
  line L60 (-20, -3) -> (-40, -3)
  line L61 (-40, -3) -> (-40, 0)
  line L62 (-40, 0) -> (-60, 0)
  line L63 (-60, 0) -> (-60, -3)
  line L64 (-60, -3) -> (-80, -3)
  line L65 (-80, -3) -> (-80, 0)
  line L66 (-80, 0) -> (-100, 0)
  line L67 (-100, 0) -> (-100, -3)
  line L68 (-100, -3) -> (-120, -3)
  line L69 (-120, -3) -> (-120, 0)
  line L70 (-120, 0) -> (-140, 0)
  line L71 (-140, 0) -> (-140, -3)
  line L72 (-140, -3) -> (-160, -3)
  line L73 (-160, -3) -> (-160, 0)
  line L74 (-160, 0) -> (-180, 0)
  line L75 (-180, 0) -> (-180, -3)
  line L76 (-180, -3) -> (-200, -3)
  line L77 (-200, -3) -> (-200, 0)
  line L78 (-200, 0) -> (-220, 0)
  line L79 (-220, 0) -> (-220, -3)
  line L80 (-220, -3) -> (-240, -3)
  line L81 (-240, -3) -> (-240, 0)
  line L82 (-240, 0) -> (-260, 0)
  line L83 (-260, 0) -> (-260, -3)
  line L84 (-260, -3) -> (-280, -3)
  line L85 (-280, -3) -> (-280, 0)
  line L86 (-280, 0) -> (-300, 0)
  line L87 (-300, 0) -> (-300, -18.5714)
  line L88 (-300, -18.5714) -> (-297, -18.5714)
  line L89 (-297, -18.5714) -> (-297, -37.1429)
  line L90 (-297, -37.1429) -> (-300, -37.1429)
  line L91 (-300, -37.1429) -> (-300, -55.7143)
  line L92 (-300, -55.7143) -> (-297, -55.7143)
  line L93 (-297, -55.7143) -> (-297, -74.2857)
  line L94 (-297, -74.2857) -> (-300, -74.2857)
  line L95 (-300, -74.2857) -> (-300, -92.8571)
sketch "TOP" plane through (0, 0, 120) normal (0, 0, 1) x (-1, 0, 0)
  line L0 (-284.4296, -73.3855) -> (-284.4296, -19.3855)
  line L1 (-284.4296, -19.3855) -> (-183.4296, -19.3855)
  line L2 (-183.4296, -19.3855) -> (-183.4296, -73.3855)
  line L3 (-183.4296, -73.3855) -> (-284.4296, -73.3855)
  line L4 (-169.4021, -72.4445) -> (-169.4021, -19.1021)
  line L5 (-169.4021, -19.1021) -> (-161.4021, -19.1021)
  line L6 (-161.4021, -19.1021) -> (-161.4021, -72.4445)
  line L7 (-161.4021, -72.4445) -> (-169.4021, -72.4445)
  line L8 (-270.7569, -113.0322) -> (-270.7569, -90.0322)
  line L9 (-270.7569, -90.0322) -> (-199.7569, -90.0322)
  line L10 (-199.7569, -90.0322) -> (-199.7569, -113.0322)
  line L11 (-199.7569, -113.0322) -> (-270.7569, -113.0322)
  circle A0 centre (-125.8569, -100.5311) radius 5
  line L12 (-151.5, -18.5714) -> (-148.5, -18.5714)
  line L13 (-148.5, -18.5714) -> (-148.5, -37.1429)
  line L14 (-148.5, -37.1429) -> (-151.5, -37.1429)
  line L15 (-151.5, -37.1429) -> (-151.5, -18.5714)
  line L16 (-151.5, -55.7143) -> (-148.5, -55.7143)
  line L17 (-148.5, -55.7143) -> (-148.5, -74.2857)
  line L18 (-148.5, -74.2857) -> (-151.5, -74.2857)
  line L19 (-151.5, -74.2857) -> (-151.5, -55.7143)
  line L20 (-151.5, -92.8571) -> (-148.5, -92.8571)
  line L21 (-148.5, -92.8571) -> (-148.5, -111.4286)
  line L22 (-148.5, -111.4286) -> (-151.5, -111.4286)
  line L23 (-151.5, -111.4286) -> (-151.5, -92.8571)
  line L24 (-300, -92.8571) -> (-297, -92.8571)
  line L25 (-297, -92.8571) -> (-297, -111.4286)
  line L26 (-297, -111.4286) -> (-300, -111.4286)
  line L27 (-300, -111.4286) -> (-300, -130)
  line L28 (-300, -130) -> (-280, -130)
  line L29 (-280, -130) -> (-280, -127)
  line L30 (-280, -127) -> (-260, -127)
  line L31 (-260, -127) -> (-260, -130)
  line L32 (-260, -130) -> (-240, -130)
  line L33 (-240, -130) -> (-240, -127)
  line L34 (-240, -127) -> (-220, -127)
  line L35 (-220, -127) -> (-220, -130)
  line L36 (-220, -130) -> (-200, -130)
  line L37 (-200, -130) -> (-200, -127)
  line L38 (-200, -127) -> (-180, -127)
  line L39 (-180, -127) -> (-180, -130)
  line L40 (-180, -130) -> (-160, -130)
  line L41 (-160, -130) -> (-160, -127)
  line L42 (-160, -127) -> (-140, -127)
  line L43 (-140, -127) -> (-140, -130)
  line L44 (-140, -130) -> (-120, -130)
  line L45 (-120, -130) -> (-120, -127)
  line L46 (-120, -127) -> (-100, -127)
  line L47 (-100, -127) -> (-100, -130)
  line L48 (-100, -130) -> (-80, -130)
  line L49 (-80, -130) -> (-80, -127)
  line L50 (-80, -127) -> (-60, -127)
  line L51 (-60, -127) -> (-60, -130)
  line L52 (-60, -130) -> (-40, -130)
  line L53 (-40, -130) -> (-40, -127)
  line L54 (-40, -127) -> (-20, -127)
  line L55 (-20, -127) -> (-20, -130)
  line L56 (-20, -130) -> (0, -130)
  line L57 (0, -130) -> (0, -111.4286)
  line L58 (0, -111.4286) -> (-3, -111.4286)
  line L59 (-3, -111.4286) -> (-3, -92.8571)
  line L60 (-3, -92.8571) -> (0, -92.8571)
  line L61 (0, -92.8571) -> (0, -74.2857)
  line L62 (0, -74.2857) -> (-3, -74.2857)
  line L63 (-3, -74.2857) -> (-3, -55.7143)
  line L64 (-3, -55.7143) -> (0, -55.7143)
  line L65 (0, -55.7143) -> (0, -37.1429)
  line L66 (0, -37.1429) -> (-3, -37.1429)
  line L67 (-3, -37.1429) -> (-3, -18.5714)
  line L68 (-3, -18.5714) -> (0, -18.5714)
  line L69 (0, -18.5714) -> (0, 0)
  line L70 (0, 0) -> (-20, 0)
  line L71 (-20, 0) -> (-20, -3)
  line L72 (-20, -3) -> (-40, -3)
  line L73 (-40, -3) -> (-40, 0)
  line L74 (-40, 0) -> (-60, 0)
  line L75 (-60, 0) -> (-60, -3)
  line L76 (-60, -3) -> (-80, -3)
  line L77 (-80, -3) -> (-80, 0)
  line L78 (-80, 0) -> (-100, 0)
  line L79 (-100, 0) -> (-100, -3)
  line L80 (-100, -3) -> (-120, -3)
  line L81 (-120, -3) -> (-120, 0)
  line L82 (-120, 0) -> (-140, 0)
  line L83 (-140, 0) -> (-140, -3)
  line L84 (-140, -3) -> (-160, -3)
  line L85 (-160, -3) -> (-160, 0)
  line L86 (-160, 0) -> (-180, 0)
  line L87 (-180, 0) -> (-180, -3)
  line L88 (-180, -3) -> (-200, -3)
  line L89 (-200, -3) -> (-200, 0)
  line L90 (-200, 0) -> (-220, 0)
  line L91 (-220, 0) -> (-220, -3)
  line L92 (-220, -3) -> (-240, -3)
  line L93 (-240, -3) -> (-240, 0)
  line L94 (-240, 0) -> (-260, 0)
  line L95 (-260, 0) -> (-260, -3)
  line L96 (-260, -3) -> (-280, -3)
  line L97 (-280, -3) -> (-280, 0)
  line L98 (-280, 0) -> (-300, 0)
  line L99 (-300, 0) -> (-300, -18.5714)
  line L100 (-300, -18.5714) -> (-297, -18.5714)
  line L101 (-297, -18.5714) -> (-297, -37.1429)
  line L102 (-297, -37.1429) -> (-300, -37.1429)
  line L103 (-300, -37.1429) -> (-300, -55.7143)
  line L104 (-300, -55.7143) -> (-297, -55.7143)
  line L105 (-297, -55.7143) -> (-297, -74.2857)
  line L106 (-297, -74.2857) -> (-300, -74.2857)
  line L107 (-300, -74.2857) -> (-300, -92.8571)
sketch "Sketch4" plane through (0, 0, 120) normal (0, 0, 1) x (-1, 0, 0)
  line L0 (-151.5, -18.5714) -> (-148.5, -18.5714)
  line L1 (-148.5, -18.5714) -> (-148.5, -37.1429)
  line L2 (-148.5, -37.1429) -> (-151.5, -37.1429)
  line L3 (-151.5, -37.1429) -> (-151.5, -18.5714)
  line L4 (-151.5, -55.7143) -> (-148.5, -55.7143)
  line L5 (-148.5, -55.7143) -> (-148.5, -74.2857)
  line L6 (-148.5, -74.2857) -> (-151.5, -74.2857)
  line L7 (-151.5, -74.2857) -> (-151.5, -55.7143)
  line L8 (-300, -55.7143) -> (-297, -55.7143)
  line L9 (-297, -55.7143) -> (-297, -74.2857)
  line L10 (-297, -74.2857) -> (-300, -74.2857)
  line L11 (-300, -111.4286) -> (-300, -130)
  line L12 (-300, -130) -> (-280, -130)
  line L13 (-280, -130) -> (-280, -127)
  line L14 (-280, -127) -> (-260, -127)
  line L15 (-260, -127) -> (-260, -130)
  line L16 (-260, -130) -> (-240, -130)
  line L17 (-240, -130) -> (-240, -127)
  line L18 (-240, -127) -> (-220, -127)
  line L19 (-220, -127) -> (-220, -130)
  line L20 (-220, -130) -> (-200, -130)
  line L21 (-200, -130) -> (-200, -127)
  line L22 (-200, -127) -> (-180, -127)
  line L23 (-180, -127) -> (-180, -130)
  line L24 (-180, -130) -> (-160, -130)
  line L25 (-160, -130) -> (-160, -127)
  line L26 (-160, -127) -> (-140, -127)
  line L27 (-140, -127) -> (-140, -130)
  line L28 (-140, -130) -> (-120, -130)
  line L29 (-120, -130) -> (-120, -127)
  line L30 (-120, -127) -> (-100, -127)
  line L31 (-100, -127) -> (-100, -130)
  line L32 (-100, -130) -> (-80, -130)
  line L33 (-80, -130) -> (-80, -127)
  line L34 (-80, -127) -> (-60, -127)
  line L35 (-60, -127) -> (-60, -130)
  line L36 (-60, -130) -> (-40, -130)
  line L37 (-40, -130) -> (-40, -127)
  line L38 (-40, -127) -> (-20, -127)
  line L39 (-20, -127) -> (-20, -130)
  line L40 (-20, -130) -> (0, -130)
  line L41 (0, -130) -> (0, -111.4286)
  line L42 (0, -74.2857) -> (-3, -74.2857)
  line L43 (-3, -74.2857) -> (-3, -55.7143)
  line L44 (-3, -55.7143) -> (0, -55.7143)
  line L45 (0, -55.7143) -> (0, -37.1429)
  line L46 (0, -37.1429) -> (-3, -37.1429)
  line L47 (-3, -37.1429) -> (-3, -18.5714)
  line L48 (-3, -18.5714) -> (0, -18.5714)
  line L49 (0, -18.5714) -> (0, 0)
  line L50 (0, 0) -> (-20, 0)
  line L51 (-20, 0) -> (-20, -3)
  line L52 (-20, -3) -> (-40, -3)
  line L53 (-40, -3) -> (-40, 0)
  line L54 (-40, 0) -> (-60, 0)
  line L55 (-60, 0) -> (-60, -3)
  line L56 (-60, -3) -> (-80, -3)
  line L57 (-80, -3) -> (-80, 0)
  line L58 (-80, 0) -> (-100, 0)
  line L59 (-100, 0) -> (-100, -3)
  line L60 (-100, -3) -> (-120, -3)
  line L61 (-120, -3) -> (-120, 0)
  line L62 (-120, 0) -> (-140, 0)
  line L63 (-140, 0) -> (-140, -3)
  line L64 (-140, -3) -> (-160, -3)
  line L65 (-160, -3) -> (-160, 0)
  line L66 (-160, 0) -> (-180, 0)
  line L67 (-180, 0) -> (-180, -3)
  line L68 (-180, -3) -> (-200, -3)
  line L69 (-200, -3) -> (-200, 0)
  line L70 (-200, 0) -> (-220, 0)
  line L71 (-220, 0) -> (-220, -3)
  line L72 (-220, -3) -> (-240, -3)
  line L73 (-240, -3) -> (-240, 0)
  line L74 (-240, 0) -> (-260, 0)
  line L75 (-260, 0) -> (-260, -3)
  line L76 (-260, -3) -> (-280, -3)
  line L77 (-280, -3) -> (-280, 0)
  line L78 (-280, 0) -> (-300, 0)
  line L79 (-300, 0) -> (-300, -18.5714)
  line L80 (-300, -18.5714) -> (-297, -18.5714)
  line L81 (-297, -18.5714) -> (-297, -37.1429)
  line L82 (-297, -37.1429) -> (-300, -37.1429)
  line L83 (-300, -37.1429) -> (-300, -55.7143)
  line L84 (-159.565, -80.1297) -> (-180.5, -80.1297)
  line L85 (-180.5, -80.1297) -> (-180.5, -19.5144)
  line L86 (-180.5, -19.5144) -> (-159.565, -19.5144)
  line L87 (-159.565, -19.5144) -> (-159.565, -80.1297)
  line L88 (-19.9408, -80.1297) -> (-129.8845, -80.1297)
  line L89 (-129.8845, -80.1297) -> (-129.8845, -19.9324)
  line L90 (-129.8845, -19.9324) -> (-19.9408, -19.9324)
  line L91 (-19.9408, -19.9324) -> (-19.9408, -80.1297)
  line L92 (-284.4296, -73.3855) -> (-284.4296, -19.3855)
  line L93 (-284.4296, -19.3855) -> (-183.4296, -19.3855)
  line L94 (-183.4296, -19.3855) -> (-183.4296, -73.3855)
  line L95 (-183.4296, -73.3855) -> (-284.4296, -73.3855)
  line L96 (-169.4021, -72.4445) -> (-169.4021, -19.1021)
  line L97 (-169.4021, -19.1021) -> (-161.4021, -19.1021)
  line L98 (-161.4021, -19.1021) -> (-161.4021, -72.4445)
  line L99 (-161.4021, -72.4445) -> (-169.4021, -72.4445)
  line L100 (-270.7569, -113.0322) -> (-270.7569, -90.0322)
  line L101 (-270.7569, -90.0322) -> (-199.7569, -90.0322)
  line L102 (-199.7569, -90.0322) -> (-199.7569, -113.0322)
  line L103 (-199.7569, -113.0322) -> (-270.7569, -113.0322)
  circle A0 centre (-125.8569, -100.5311) radius 5
  line L104 (-151.5, -92.8571) -> (-148.5, -92.8571)
  line L105 (-148.5, -92.8571) -> (-148.5, -111.4286)
  line L106 (-148.5, -111.4286) -> (-151.5, -111.4286)
  line L107 (-151.5, -111.4286) -> (-151.5, -92.8571)
  line L108 (-300, -92.8571) -> (-297, -92.8571)
  line L109 (-297, -92.8571) -> (-297, -111.4286)
  line L110 (-297, -111.4286) -> (-300, -111.4286)
  line L111 (0, -111.4286) -> (-3, -111.4286)
  line L112 (-3, -111.4286) -> (-3, -92.8571)
  line L113 (-3, -92.8571) -> (0, -92.8571)
  line L114 (0, -92.8571) -> (0, -74.2857)
  line L115 (-300, -74.2857) -> (-300, -92.8571)
  constraint horizontal L84
  constraint vertical L85
  constraint horizontal L86
  constraint vertical L87
  constraint horizontal L88
  constraint vertical L89
  constraint horizontal L90
  constraint vertical L91
extrude "Extrude3" [rolled back] taper angle 0
sketch "Sketch6" plane through (148.5, 0, 0) normal (-1, 0, 0) x (0, -1, 0)
  line L0 (-3, 117) -> (-18.5714, 117)
  line L1 (-18.5714, 117) -> (-18.5714, 120)
  line L2 (-18.5714, 120) -> (-37.1429, 120)
  line L3 (-37.1429, 120) -> (-37.1429, 117)
  line L4 (-37.1429, 117) -> (-55.7143, 117)
  line L5 (-55.7143, 117) -> (-55.7143, 120)
  line L6 (-55.7143, 120) -> (-74.2857, 120)
  line L7 (-74.2857, 120) -> (-74.2857, 117)
  line L8 (-74.2857, 117) -> (-92.8571, 117)
  line L9 (-127, 117) -> (-127, 96.6)
  line L10 (-127, 96.6) -> (-130, 96.6)
  line L11 (-130, 96.6) -> (-130, 73.2)
  line L12 (-130, 73.2) -> (-127, 73.2)
  line L13 (-127, 73.2) -> (-127, 49.8)
  line L14 (-127, 49.8) -> (-130, 49.8)
  line L15 (-130, 49.8) -> (-130, 26.4)
  line L16 (-130, 26.4) -> (-127, 26.4)
  line L17 (-127, 26.4) -> (-127, 3)
  line L18 (-127, 3) -> (-111.4286, 3)
  line L19 (-74.2857, 3) -> (-74.2857, 0)
  line L20 (-111.4286, 0) -> (-92.8571, 0)
  line L21 (-55.7143, 0) -> (-55.7143, 3)
  line L22 (-55.7143, 3) -> (-37.1429, 3)
  line L23 (-37.1429, 3) -> (-37.1429, 0)
  line L24 (-37.1429, 0) -> (-18.5714, 0)
  line L25 (-18.5714, 0) -> (-18.5714, 3)
  line L26 (-18.5714, 3) -> (-3, 3)
  line L27 (-3, 3) -> (-3, 26.4)
  line L28 (-3, 26.4) -> (0, 26.4)
  line L29 (0, 26.4) -> (0, 49.8)
  line L30 (0, 49.8) -> (-3, 49.8)
  line L31 (-3, 49.8) -> (-3, 73.2)
  line L32 (-3, 73.2) -> (0, 73.2)
  line L33 (0, 73.2) -> (0, 96.6)
  line L34 (0, 96.6) -> (-3, 96.6)
  line L35 (-3, 96.6) -> (-3, 117)
  line L36 (-90.428, 89.969) -> (-7.9498, 89.969)
  line L37 (-7.9498, 89.969) -> (-7.9498, 75.2472)
  line L38 (-7.9498, 75.2472) -> (-90.428, 75.2472)
  line L39 (-90.428, 75.2472) -> (-90.428, 89.969)
  circle A0 centre (-63.791, 90.8075) radius 9.4231
  line L40 (-92.8571, 117) -> (-92.8571, 120)
  line L41 (-92.8571, 120) -> (-111.4286, 120)
  line L42 (-111.4286, 120) -> (-111.4286, 117)
  line L43 (-111.4286, 117) -> (-127, 117)
  line L44 (-111.4286, 3) -> (-111.4286, 0)
  line L45 (-92.8571, 0) -> (-92.8571, 3)
  line L46 (-92.8571, 3) -> (-74.2857, 3)
  line L47 (-74.2857, 0) -> (-55.7143, 0)
  constraint horizontal L36
  constraint vertical L37
  constraint horizontal L38
  constraint vertical L39
extrude "Extrude9" [rolled back] taper angle 0 in component "Main Box"
sketch "FRONTBACK (2)" plane through (0, 0, 0) normal (0, -1, 0) x (1, 0, 0)
  line L0 (151.5, 26.4) -> (148.5, 26.4)
  line L1 (148.5, 26.4) -> (148.5, 49.8)
  line L2 (148.5, 49.8) -> (151.5, 49.8)
  line L3 (151.5, 49.8) -> (151.5, 26.4)
  line L4 (151.5, 73.2) -> (148.5, 73.2)
  line L5 (148.5, 73.2) -> (148.5, 96.6)
  line L6 (148.5, 96.6) -> (151.5, 96.6)
  line L7 (151.5, 96.6) -> (151.5, 73.2)
  line L8 (300, 117) -> (280, 117)
  line L9 (280, 117) -> (280, 120)
  line L10 (280, 120) -> (260, 120)
  line L11 (260, 120) -> (260, 117)
  line L12 (260, 117) -> (240, 117)
  line L13 (240, 117) -> (240, 120)
  line L14 (240, 120) -> (220, 120)
  line L15 (220, 120) -> (220, 117)
  line L16 (220, 117) -> (200, 117)
  line L17 (200, 117) -> (200, 120)
  line L18 (200, 120) -> (180, 120)
  line L19 (180, 120) -> (180, 117)
  line L20 (180, 117) -> (160, 117)
  line L21 (160, 117) -> (160, 120)
  line L22 (160, 120) -> (140, 120)
  line L23 (140, 120) -> (140, 117)
  line L24 (140, 117) -> (120, 117)
  line L25 (120, 117) -> (120, 120)
  line L26 (120, 120) -> (100, 120)
  line L27 (100, 120) -> (100, 117)
  line L28 (100, 117) -> (80, 117)
  line L29 (80, 117) -> (80, 120)
  line L30 (80, 120) -> (60, 120)
  line L31 (60, 120) -> (60, 117)
  line L32 (60, 117) -> (40, 117)
  line L33 (40, 117) -> (40, 120)
  line L34 (40, 120) -> (20, 120)
  line L35 (20, 120) -> (20, 117)
  line L36 (20, 117) -> (0, 117)
  line L37 (0, 117) -> (0, 96.6)
  line L38 (0, 96.6) -> (3, 96.6)
  line L39 (3, 96.6) -> (3, 73.2)
  line L40 (3, 73.2) -> (0, 73.2)
  line L41 (0, 73.2) -> (0, 49.8)
  line L42 (0, 49.8) -> (3, 49.8)
  line L43 (3, 49.8) -> (3, 26.4)
  line L44 (3, 26.4) -> (0, 26.4)
  line L45 (0, 26.4) -> (0, 3)
  line L46 (0, 3) -> (20, 3)
  line L47 (20, 3) -> (20, 0)
  line L48 (20, 0) -> (40, 0)
  line L49 (40, 0) -> (40, 3)
  line L50 (40, 3) -> (60, 3)
  line L51 (60, 3) -> (60, 0)
  line L52 (60, 0) -> (80, 0)
  line L53 (80, 0) -> (80, 3)
  line L54 (80, 3) -> (100, 3)
  line L55 (100, 3) -> (100, 0)
  line L56 (100, 0) -> (120, 0)
  line L57 (120, 0) -> (120, 3)
  line L58 (120, 3) -> (140, 3)
  line L59 (140, 3) -> (140, 0)
  line L60 (140, 0) -> (160, 0)
  line L61 (160, 0) -> (160, 3)
  line L62 (160, 3) -> (180, 3)
  line L63 (180, 3) -> (180, 0)
  line L64 (180, 0) -> (200, 0)
  line L65 (200, 0) -> (200, 3)
  line L66 (200, 3) -> (220, 3)
  line L67 (220, 3) -> (220, 0)
  line L68 (220, 0) -> (240, 0)
  line L69 (240, 0) -> (240, 3)
  line L70 (240, 3) -> (260, 3)
  line L71 (260, 3) -> (260, 0)
  line L72 (260, 0) -> (280, 0)
  line L73 (280, 0) -> (280, 3)
  line L74 (280, 3) -> (300, 3)
  line L75 (300, 3) -> (300, 26.4)
  line L76 (300, 26.4) -> (297, 26.4)
  line L77 (297, 26.4) -> (297, 49.8)
  line L78 (297, 49.8) -> (300, 49.8)
  line L79 (300, 49.8) -> (300, 73.2)
  line L80 (300, 73.2) -> (297, 73.2)
  line L81 (297, 73.2) -> (297, 96.6)
  line L82 (297, 96.6) -> (300, 96.6)
  line L83 (300, 96.6) -> (300, 117)
sketch "LEFTRIGHT" plane through (0, 0, 0) normal (-1, 0, 0) x (0, -1, 0)
  line L0 (-3, 117) -> (-18.5714, 117)
  line L1 (-18.5714, 117) -> (-18.5714, 120)
  line L2 (-18.5714, 120) -> (-37.1429, 120)
  line L3 (-37.1429, 120) -> (-37.1429, 117)
  line L4 (-37.1429, 117) -> (-55.7143, 117)
  line L5 (-55.7143, 117) -> (-55.7143, 120)
  line L6 (-55.7143, 120) -> (-74.2857, 120)
  line L7 (-74.2857, 120) -> (-74.2857, 117)
  line L8 (-74.2857, 117) -> (-92.8571, 117)
  line L9 (-127, 117) -> (-127, 96.6)
  line L10 (-127, 96.6) -> (-130, 96.6)
  line L11 (-130, 96.6) -> (-130, 73.2)
  line L12 (-130, 73.2) -> (-127, 73.2)
  line L13 (-127, 73.2) -> (-127, 49.8)
  line L14 (-127, 49.8) -> (-130, 49.8)
  line L15 (-130, 49.8) -> (-130, 26.4)
  line L16 (-130, 26.4) -> (-127, 26.4)
  line L17 (-127, 26.4) -> (-127, 3)
  line L18 (-127, 3) -> (-111.4286, 3)
  line L19 (-74.2857, 3) -> (-74.2857, 0)
  line L20 (-111.4286, 0) -> (-92.8571, 0)
  line L21 (-55.7143, 0) -> (-55.7143, 3)
  line L22 (-55.7143, 3) -> (-37.1429, 3)
  line L23 (-37.1429, 3) -> (-37.1429, 0)
  line L24 (-37.1429, 0) -> (-18.5714, 0)
  line L25 (-18.5714, 0) -> (-18.5714, 3)
  line L26 (-18.5714, 3) -> (-3, 3)
  line L27 (-3, 3) -> (-3, 26.4)
  line L28 (-3, 26.4) -> (0, 26.4)
  line L29 (0, 26.4) -> (0, 49.8)
  line L30 (0, 49.8) -> (-3, 49.8)
  line L31 (-3, 49.8) -> (-3, 73.2)
  line L32 (-3, 73.2) -> (0, 73.2)
  line L33 (0, 73.2) -> (0, 96.6)
  line L34 (0, 96.6) -> (-3, 96.6)
  line L35 (-3, 96.6) -> (-3, 117)
  line L36 (-92.8571, 117) -> (-92.8571, 120)
  line L37 (-92.8571, 120) -> (-111.4286, 120)
  line L38 (-111.4286, 120) -> (-111.4286, 117)
  line L39 (-111.4286, 117) -> (-127, 117)
  line L40 (-111.4286, 3) -> (-111.4286, 0)
  line L41 (-92.8571, 0) -> (-92.8571, 3)
  line L42 (-92.8571, 3) -> (-74.2857, 3)
  line L43 (-74.2857, 0) -> (-55.7143, 0)